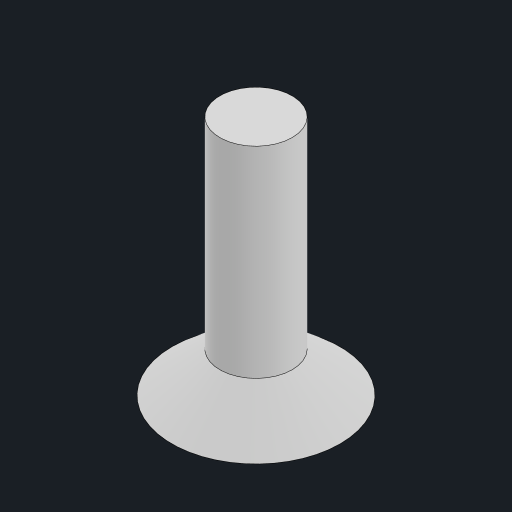
# Autodesk Inventor part: neji
Saved by Autodesk Inventor 2023 (Build 270158000, 158)
## iProperties
Created: 2022-06-21
Part Number: neji
Material: Generic
Document SubType Name: Modeling
Designer: legot
Density: 1 g/cm^3
Appearance: Default
Author: legot
Autodesk Inventor part; units mm, degrees
ref_plane "YZ Plane" through (0, 0, 0) normal (1, 0, 0) x (0, 1, 0)
ref_plane "XZ Plane" through (0, 0, 0) normal (0, 1, 0) x (-1, 0, 0)
ref_plane "XY Plane" through (0, 0, 0) normal (0, 0, 1) x (1, 0, 0)
sketch "スケッチ1" plane through (0, 0, 0) normal (0, 0, 1) x (1, 0, 0)
  line L0 (0, 0) -> (0.9, 0)
  line L1 (0.9, 0) -> (0.9, 6)
  line L2 (0.9, 6) -> (0, 6)
  line L3 (0, 6) -> (0, 0)
  line L4 (0.9, 0) -> (2.0918, 0)
  line L5 (2.0918, 0) -> (0.9, 1)
  dimension "d0" = 0.9
  dimension "d1" = 40
  dimension "d2" = 1
  dimension "d3" = 5
  constraints: 12 end point, 2 horizontal, 2 parallel, 1 perpendicular, 1 point on line
  measures "d0" distance of L0.start L0.end
  measures "d1" angle of L4 L5
  measures "d2" distance from line of L4 L5.end
  measures "d3" distance of L1.end L5.end
revolve "回転1" add sketch "スケッチ1" angle 360 about axis through (0, 6, 0) along (0, -1, 0)
